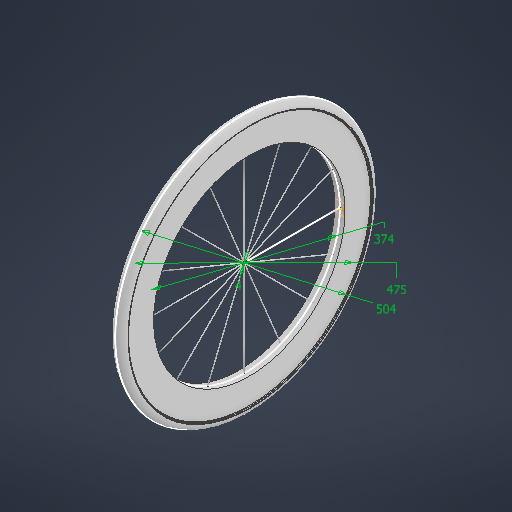
# Autodesk Inventor part: wheel
Saved by Autodesk Inventor 2026.3 (Build 303398000, 398)
## iProperties
Created: 2026-08-06
Part Number: wheel
Material: 일반
Document SubType Name: Modeling
Designer: hojin
Density: 1 g/cm^3
Appearance: 기본값
Author: hojin
Autodesk Inventor part; units mm, degrees
ref_plane "YZ Plane" through (0, 0, 0) normal (1, 0, 0) x (0, 1, 0)
ref_plane "XZ Plane" through (0, 0, 0) normal (0, 1, 0) x (-1, 0, 0)
ref_plane "XY Plane" through (0, 0, 0) normal (0, 0, 1) x (1, 0, 0)
sketch "스케치1" plane through (0, 0, 0) normal (1, 0, 0) x (0, 1, 0)
  circle A0 centre (0, 0) radius 252
  circle A1 centre (0, 0) radius 237.5
  circle A2 centre (0, 0) radius 187
  line L0 (0, -187) -> (0, 0)
  circle A3 centre (0, 0) radius 2
  dimension "d2" = 374
  dimension "d0" = 504
  dimension "d1" = 475
  dimension "d26" = 4
  constraints: 3 centre point, 3 coincident, 2 end point, 1 concentric, 1 vertical, 1 vertical alignment, 2 other
  measures "d0" diameter of A0
  measures "d1" diameter of A1
  measures "d26" diameter of A3
extrude "돌출1" add sketch "스케치1" along normal mid plane 20 contours A1
extrude "돌출2" add sketch "스케치1" along normal mid plane 25 contours A0
fillet "모깎기1" radius 12.5 2 edges at (-12.5, -252, 0) (12.5, -252, 0)
ref_plane "작업 평면1" through (0, 0, -187) normal (0, 0, 1) x (1, 0, 0)
sketch "스케치2" plane through (0, 0, -187) normal (0, 0, 1) x (1, 0, 0)
  circle A0 centre (0, 0) radius 1
  dimension "d12" = 2
  constraints: 1 centre point, 1 coincident
  measures "d12" diameter of A0
sweep "스윕1" add profiles "스케치2" path "스케치1" path curves L0
pattern_circular "원형 패턴1" count 16 over 360 about axis through (-10, 0, 0) along (1, 0, 0) of "스윕1"
fillet "모깎기2" radius 1 2 edges at (12.5, -237.5, 0) (10, -237.5, 0)
hole "구멍1" at (0, 0, 0) direction (1, 0, 0) diameter 4 end through all both
sketch "스케치3" plane through (0, 0, -187) normal (0, 0, 1) x (1, 0, 0)
  point P0 (0, 0)
